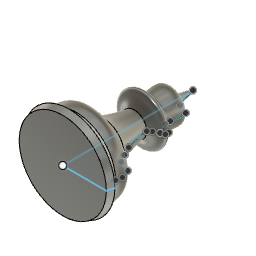
test_pawn (Autodesk Fusion 360 design; units mm, degrees)
Autodesk Fusion 360 part; units mm, degrees
sketch "Sketch1" plane through (0, 0, 0) normal (0, 0, 1) x (1, 0, 0)
  line L0 (1.778, 0.254) -> (1.5288, 0.531)
  spline S0 degree 5 poles (0.4791, 2.7948) (0.4799, 2.7956) (0.4829, 2.7985) (0.4915, 2.8067) (0.5108, 2.8247) (0.5451, 2.8553) (0.5857, 2.8895) (0.6293, 2.9229) (0.6734, 2.952) (0.7169, 2.9748) (0.7595, 2.9909) (0.8009, 3.001) (0.8409, 3.0076) (0.8787, 3.0146) (0.9131, 3.0263) (0.9425, 3.0457) (0.9648, 3.0741) (0.9776, 3.1088) (0.9786, 3.1448) (0.9663, 3.1766) (0.9403, 3.2002) (0.9023, 3.2157) (0.8559, 3.2268) (0.8056, 3.2387) (0.7556, 3.2562) (0.7097, 3.2819) (0.6699, 3.3141) (0.6369, 3.3488) (0.6111, 3.3819) (0.5921, 3.411) (0.5804, 3.4382) (0.5769, 3.4703) (0.582, 3.5155) (0.5954, 3.5807) (0.6154, 3.6686) (0.638, 3.7747) (0.6577, 3.8888) (0.6686, 3.9985) (0.6651, 4.0916) (0.6432, 4.1588) (0.6015, 4.1964) (0.5418, 4.2099) (0.4695, 4.2125) (0.3913, 4.2207) (0.3146, 4.2509) (0.2456, 4.3155) (0.1885, 4.4189) (0.1438, 4.554) (0.1096, 4.7062) (0.0824, 4.8559) (0.058, 4.9826) (0.0373, 5.0501) (0.0196, 5.0756) (0.0067, 5.0805) (0, 5.08) knots 0 0 0 0 0 0 0.02 0.04 0.06 0.08 0.1 0.12 0.14 0.16 0.18 0.2 0.22 0.24 0.26 0.28 0.3 0.32 0.34 0.36 0.38 0.4 0.42 0.44 0.46 0.48 0.5 0.52 0.54 0.56 0.58 0.6 0.62 0.64 0.66 0.68 0.7 0.72 0.74 0.76 0.78 0.8 0.82 0.84 0.86 0.88 0.9 0.92 0.94 0.96 0.98 1 1 1 1 1 1
  line L1 (0.3338, 2.6448) -> (0.6244, 2.9447)
  line L2 (0.2903, 5.1024) -> (-0.2903, 5.0576)
  line L3 (0, 0) -> (0, 5.08)
  line L4 (1.6981, 0) -> (1.778, 0.254)
  spline S1 degree 5 poles (1.5288, 0.531) (1.5291, 0.5327) (1.5303, 0.5385) (1.534, 0.5536) (1.5422, 0.5866) (1.555, 0.6458) (1.5667, 0.7182) (1.573, 0.7983) (1.5698, 0.8796) (1.5537, 0.9556) (1.5223, 1.021) (1.4745, 1.0724) (1.411, 1.1092) (1.3343, 1.1351) (1.2493, 1.1573) (1.1616, 1.1838) (1.0774, 1.2219) (1.0021, 1.2756) (0.9401, 1.3436) (0.8937, 1.4175) (0.8635, 1.4861) (0.8482, 1.5381) (0.8447, 1.5663) (0.8482, 1.5709) (0.8523, 1.5615) (0.8506, 1.5519) (0.8386, 1.5567) (0.8145, 1.5859) (0.7797, 1.6453) (0.7368, 1.7366) (0.6898, 1.8579) (0.6425, 2.0035) (0.5981, 2.1645) (0.5587, 2.3298) (0.5261, 2.4873) (0.5013, 2.6251) (0.4881, 2.7116) (0.4821, 2.76) (0.4798, 2.7845) (0.4791, 2.7948) knots 0 0 0 0 0 0 0.028571 0.057143 0.085714 0.114286 0.142857 0.171429 0.2 0.228571 0.257143 0.285714 0.314286 0.342857 0.371429 0.4 0.428571 0.457143 0.485714 0.514286 0.542857 0.571429 0.6 0.628571 0.657143 0.685714 0.714286 0.742857 0.771429 0.8 0.828571 0.857143 0.885714 0.914286 0.942857 0.971429 1 1 1 1 1 1
  line L5 (1.4887, 0.3032) -> (1.5689, 0.7588)
  line L6 (0.5134, 2.2949) -> (0.4447, 3.2946)
  line L7 (0, 0) -> (1.6981, 0)
  point P0 (0.8, 3)
  point P1 (1.4426, 1.0883)
  point P2 (0.6791, 1.8948)
  point P3 (0.6, 3.6)
  point P4 (1.5689, 0.7588)
  point P5 (0.6238, 4.1705)
  point P6 (1.016, 1.27)
  point P7 (0.6, 2.9)
  point P8 (0.6, 3.4)
  point P9 (0.254, 4.318)
  point P10 (0.7544, 3.2592)
  point P11 (0.9531, 3.186)
  point P12 (0.8468, 1.5554)
  point P13 (0.9479, 3.0552)
  point P14 (0.8468, 1.5554)
  constraint midpoint L0.end L5
  constraint coincident P14 P12
  constraint midpoint S0.start L1
  constraint midpoint S0.start L6
  constraint coincident P4 L5.end
revolve "Revolve1" add sketch "Sketch1" angle 360 about axis through (0, 0, 0) along (0, 1, 0)
